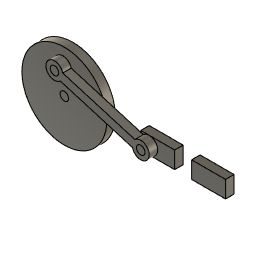
motor_pushing_block (Autodesk Fusion 360 design; units mm, degrees)
Autodesk Fusion 360 part; units mm, degrees
sketch "Sketch1" plane through (0, 0, 0) normal (0, 1, 0) x (1, 0, 0)
  circle A0 centre (0, 0) radius 25
  circle A1 centre (-0.8514, -15.1494) radius 2.5
  line L0 (65, 5) -> (45, 5)
  line L1 (45, 5) -> (65, 5)
  line L2 (65, 5) -> (65, -5)
  line L3 (65, -5) -> (45, -5)
  line L4 (45, -5) -> (45, 5)
  circle A2 centre (50.0137, 0) radius 2.5
  circle A3 centre (-0.8514, -15.1494) radius 5
  circle A4 centre (50.0137, 0) radius 5
  line L5 (49.3001, 2.396) -> (-1.565, -12.7534)
  line L6 (50.7273, -2.396) -> (-0.1378, -17.5454)
  circle A5 centre (0, 0) radius 2.5
  line L7 (75, -5) -> (95, -5)
  line L8 (95, -5) -> (95, 5)
  line L9 (95, 5) -> (75, 5)
  line L10 (75, 5) -> (75, -5)
  dimension "d1" = 50
  dimension "d2" = 5
  dimension "d3" = 5
  dimension "d4" = 10
  dimension "d5" = 10
  dimension "d6" = 5
  constraint coincident A0.centre A5.centre
  constraint horizontal L0
  constraint horizontal L1
  constraint vertical L2
  constraint horizontal L3
  constraint vertical L4
  constraint concentric A1 A3
  constraint concentric A2 A4
  constraint coincident A2 L5.start
  constraint coincident A1 L5.end
  constraint tangent A1 L5
  constraint tangent A2 L5
  constraint coincident A2 L6.start
  constraint coincident A1 L6.end
  constraint tangent A1 L6
  constraint tangent A2 L6
  constraint coincident L0.start L1.end
  constraint concentric A0 A5
  constraint horizontal L7
  constraint vertical L8
  constraint horizontal L9
  constraint vertical L10
  measures "d1" diameter of A0
  measures "d2" diameter of A1
  measures "d3" diameter of A2
  measures "d4" diameter of A3
  measures "d5" diameter of A4
  measures "d6" diameter of A5
extrude "Extrude1" add sketch "Sketch1" along normal blind 5 contours A0 A3 L5 L6 | A0 A3 L5 L6 | A1 A3 L5 L6 | A1 A3 L5 L6 | A1 makes body 1 in component "wheel"
extrude "Extrude2" add sketch "Sketch1" against normal blind 5 separate body contours A1 makes body 2 in component "wheel"
extrude "Extrude1'" add sketch "Sketch1" along normal blind 5 separate body contours L3 L4 A4 L6 | L4 A4 L5 L6 | L0 L1 L4 A4 L5 | A2 A4 L5 L6 | A2 A4 L5 L6 | L0 L1 L2 L3 A4 | A2 makes body 3 in component "block1"
extrude "Extrude2'" add sketch "Sketch1" against normal blind 5 contours A2 bodies 3 in component "block1"
extrude "Extrude1''" add sketch "Sketch1" against normal blind 5 separate body contours A0 A3 L5 L6 | A0 L4 L5 L6 | L4 A4 L5 L6 | A1 A3 L5 L6 | A1 A3 L5 L6 | A2 A4 L5 L6 | A2 A4 L5 L6 picked at (17.0297, -7.8277) makes body 4 in component "arm"
extrude "Extrude1'''" add sketch "Sketch1" along normal blind 5 separate body contours L7 L8 L9 L10 makes body 5 in component "block2\\"
extrude "Extrude1''''" add sketch "Sketch1" along normal blind 10 separate body contours A5 makes body 6 in component "ground"
component "wheel" placed x (1, 0, 0) y (0, 1, 0) z (0, 0, 1) at (0, 0, 0)
component "block1" placed x (1, 0, 0) y (0, 1, 0) z (0, 0, 1) at (0, 0, 0)
component "arm" placed x (1, 0, 0) y (0, 1, 0) z (0, 0, 1) at (0, 0, 0)
component "block2\\" placed x (1, 0, 0) y (0, 1, 0) z (0, 0, 1) at (0, 0, 0)
component "ground" placed x (1, 0, 0) y (0, 1, 0) z (0, 0, 1) at (0, 0, 0)
